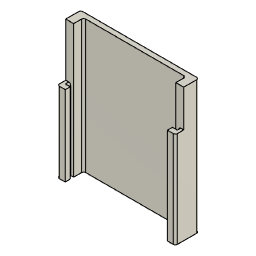
Piunora-Bottom-Protector v6 (Autodesk Fusion 360 design; units mm, degrees)
Autodesk Fusion 360 part; units mm, degrees
sketch "Sketch1" plane through (0, 0, 0) normal (0, 1, 0) x (1, 0, 0)
  line L0 (27, -5) -> (-27, -5)
  line L1 (-27, -5) -> (-27, 5)
  line L2 (-27, 5) -> (27, 5)
  line L3 (27, 5) -> (27, -5)
  line L4 (27, -5) -> (-27, 5) construction
  line L5 (-27, -5) -> (27, 5) construction
  line L6 (-29.5, -1.7) -> (29.5, -1.7)
  line L7 (29, 0) -> (-28, 0) construction
  line L8 (29.5, 7.5) -> (29.5, -7.5)
  line L9 (29.5, -7.5) -> (-29.5, -7.5)
  line L10 (-29.5, -7.5) -> (-29.5, 7.5)
  line L11 (-29.5, 7.5) -> (29.5, 7.5)
  line L12 (-27, 0) -> (-25.55, 0)
  line L13 (-25.55, 0) -> (-25.55, 5)
  line L14 (0, -10.5) -> (0, 11)
  line L15 (-29.5, -4.2) -> (-25.55, -4.2)
  line L16 (-25.55, -4.2) -> (-25.55, -1.7)
  line L17 (29.5, -4.2) -> (25.55, -4.2)
  line L18 (25.55, -4.2) -> (25.55, -1.7)
  line L19 (25.55, 0) -> (25.55, 5)
  line L20 (27, 0) -> (25.55, 0)
  dimension "d1" = 54
  dimension "d2" = 10
  dimension "d3" = 1.7
  dimension "d4" = -2.5
  dimension "d5" = 1.45
  dimension "d6" = 3.95
  dimension "d7" = 2.5
  constraint horizontal L0
  constraint perpendicular L0 L1
  constraint parallel L0 L2
  constraint parallel L1 L3
  constraint coincident L4 origin
  constraint coincident L5 origin
  constraint perpendicular L3 L6
  constraint perpendicular L1 L7
  constraint coincident L6.start L10
  constraint coincident L6.end L8
  constraint midpoint L1 L12.start
  constraint perpendicular L1 L12
  constraint coincident L2 L13.end
  constraint perpendicular L2 L13
  constraint perpendicular L11 L14
  constraint coincident L10 L15.start
  constraint perpendicular L10 L15
  constraint coincident L6 L16.end
  constraint perpendicular L6 L16
  constraint symmetric L12.start L14 L20.start
  constraint symmetric L12.end L14 L19.start
  constraint symmetric L13.end L14 L19.end
  constraint symmetric L14 L15.start L17.start
  constraint symmetric L14 L15.end L17.end
  constraint symmetric L14 L16.end L18.end
  measures "d1" distance of L1.end L2.end
  measures "d2" distance of L0.end L1.end
  measures "d3" distance of L6 L7
  measures "d5" distance of L12.start L12.end
  measures "d6" distance of L15.start L15.end
  measures "d7" distance of L6 L15
extrude "Extrude1" add sketch "Sketch1" along normal blind 66.5 contours L3 L6 L17 L18 | L3 L6 L8 L17 | L2 L3 L6 L8 L11 L14 | L1 L6 L10 L15 | L1 L6 L15 L16 | L1 L2 L6 L10 L11 L14 | L2 L3 L19 L20 | L1 L2 L12 L13
sketch "Sketch2" plane through (0, 0, 4.2) normal (0, 0, 1) x (-1, 0, 0)
  line L0 (-25.55, 0) -> (-29.5, 0)
  line L1 (-29.5, 0) -> (-29.5, -66.5)
  line L2 (-29.5, -66.5) -> (-25.55, -66.5)
  line L3 (-25.55, -66.5) -> (-25.55, 0)
  line L4 (-29.5, -66.5) -> (-22.52, -66.5)
  line L5 (-22.52, -66.5) -> (-22.52, -48)
  line L6 (-22.52, -48) -> (-29.5, -48)
  line L7 (-29.5, -48) -> (-29.5, -66.5)
  line L8 (30.3302, -66.5) -> (24.9629, -66.5)
  line L9 (24.9629, -66.5) -> (24.9629, -40)
  line L10 (24.9629, -40) -> (30.3302, -40)
  line L11 (30.3302, -40) -> (30.3302, -66.5)
  dimension "d10" = 18.5
  dimension "d11" = 26.5
  constraint horizontal L4
  constraint vertical L5
  constraint horizontal L6
  constraint vertical L7
  constraint coincident L1.end L2.start
  constraint horizontal L8
  constraint vertical L9
  constraint horizontal L10
  constraint vertical L11
  measures "d10" distance of L1.end L6.end
  measures "d11" distance of L8.start L10.end
extrude "Extrude2" cut sketch "Sketch2" against normal up to surface (4.2 mm away) contours L1 L2 L3 L4 L6 L7 | L8 L9 L10 L11
fillet "Fillet1" radius 1 8 edges at (-29.5, 20, 4.2) (29.5, 24, 4.2) (-29.5, 33.25, -7.5) (29.5, 33.25, -7.5) (25.55, 33.25, -5) (-25.55, 33.25, -5) (27, 48, 0.85) (-27, 40, 0.85)
move_body "Move1" bodies 1 to x (1, 0, 0) y (0, 0, 1) z (0, -1, 0) at (0, -7.5, -7.5)
equation "d6 = 2.5 mm + 1.45 mm"
